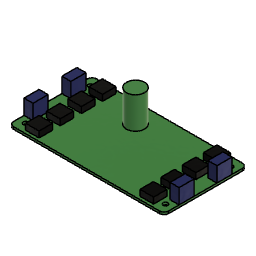
四路驱动模块 v2 (Autodesk Fusion 360 design; units mm, degrees)
Autodesk Fusion 360 part; units mm, degrees
sketch "草图1" plane through (0, 0, 0) normal (0, 0, 1) x (1, 0, 0)
  line L0 (3, 0) -> (100.2, 0)
  line L1 (103.2, 3) -> (103.2, 52.2)
  line L2 (100.2, 55.2) -> (3, 55.2)
  line L3 (0, 52.2) -> (0, 3)
  line L4 (-10, 27.6) -> (117.08, 27.6)
  line L5 (51.6, 65) -> (51.6, -15)
  circle A0 centre (5, 49.2) radius 1.6
  circle A1 centre (98.2, 49.2) radius 1.6
  circle A2 centre (5, 6) radius 1.6
  circle A3 centre (98.2, 6) radius 1.6
  arc A4 (3, 55.2) -> (0, 52.2) centre (3, 52.2) ccw
  arc A5 (103.2, 52.2) -> (100.2, 55.2) centre (100.2, 52.2) ccw
  arc A6 (100.2, 0) -> (103.2, 3) centre (100.2, 3) ccw
  arc A7 (0, 3) -> (3, 0) centre (3, 3) ccw
  point P0 (103.2, 0)
  point P1 (0, 55.2)
  dimension "d1" = 103.2
  dimension "d2" = 55.2
  dimension "d3" = 3.2
  dimension "d4" = 93.2
  dimension "d5" = 43.2
  dimension "d6" = 3
  constraint horizontal L0
  constraint vertical L1
  constraint horizontal L2
  constraint vertical L3
  constraint perpendicular L1 L4
  constraint perpendicular L2 L5
  constraint symmetric L1 L3 L5
  constraint symmetric L0 L2 L4
  constraint symmetric L5 A0 A1
  constraint symmetric L4 A0 A2
  constraint symmetric L4 A1 A3
  constraint coincident P1 L2
  constraint coincident P1 L3
  constraint tangent L2 A4
  constraint tangent L3 A4
  constraint tangent L1 A5
  constraint tangent L2 A5
  constraint equal A4 A5
  constraint coincident P0 L0
  constraint coincident P0 L1
  constraint tangent L0 A6
  constraint tangent L1 A6
  constraint equal A4 A6
  constraint tangent L0 A7
  constraint tangent L3 A7
  constraint equal A4 A7
  measures "d1" distance of origin P0
  measures "d2" distance of origin P1
  measures "d3" diameter of A0
  measures "d4" distance of A2.centre A3.centre
  measures "d5" distance of A0.centre A2.centre
  measures "d6" radius of A4
extrude "拉伸1" add sketch "草图1" along normal blind 1.5 makes body 1
sketch "草图2" plane through (0, 0, 1.5) normal (0, 0, 1) x (-1, 0, 0)
  circle A0 centre (-98.2, -6) radius 1.6
  circle A1 centre (-5, -49.2) radius 1.6
  circle A2 centre (-5, -6) radius 1.6
  circle A3 centre (-98.2, -49.2) radius 1.6
  arc A4 (0, -3) -> (-3, 0) centre (-3, -3) ccw
  line L0 (-3, 0) -> (-100.2, 0)
  arc A5 (-100.2, 0) -> (-103.2, -3) centre (-100.2, -3) ccw
  line L1 (-103.2, -3) -> (-103.2, -52.2)
  arc A6 (-103.2, -52.2) -> (-100.2, -55.2) centre (-100.2, -52.2) ccw
  line L2 (-100.2, -55.2) -> (-3, -55.2)
  arc A7 (-3, -55.2) -> (0, -52.2) centre (-3, -52.2) ccw
  line L3 (0, -52.2) -> (0, -3)
  line L4 (11.7384, -27.6) -> (-122.0621, -27.6)
  line L5 (-51.6, -62.4053) -> (-51.6, 35)
  line L6 (0, -45.2) -> (-6, -45.2)
  line L7 (-6, -45.2) -> (-6, -35.2)
  line L8 (-6, -35.2) -> (0, -35.2)
  line L9 (0, -35.2) -> (0, -45.2)
  line L10 (-97.2, -35.2) -> (-103.2, -35.2)
  line L11 (-103.2, -35.2) -> (-103.2, -45.2)
  line L12 (-103.2, -45.2) -> (-97.2, -45.2)
  line L13 (-97.2, -45.2) -> (-97.2, -35.2)
  line L14 (0, -10) -> (-6, -10)
  line L15 (-6, -10) -> (-6, -20)
  line L16 (0, -20) -> (0, -10)
  line L17 (-6, -20) -> (0, -20)
  line L18 (-97.2, -20) -> (-103.2, -20)
  line L19 (-103.2, -10) -> (-97.2, -10)
  line L20 (-97.2, -10) -> (-97.2, -20)
  line L21 (-103.2, -20) -> (-103.2, -10)
  dimension "d9" = 10
  dimension "d10" = 6
  dimension "d11" = 10
  constraint perpendicular L3 L4
  constraint vertical L5
  constraint symmetric L1 L3 L5
  constraint symmetric L0 L2 L4
  constraint horizontal L6
  constraint vertical L7
  constraint horizontal L8
  constraint vertical L9
  constraint coincident L3 L6.start
  constraint symmetric L5 L6.start L11.end
  constraint symmetric L5 L6.end L12.end
  constraint symmetric L5 L7.end L10.start
  constraint symmetric L5 L8.end L10.end
  constraint symmetric L4 L6.start L14.start
  constraint symmetric L4 L6.end L14.end
  constraint symmetric L4 L7.end L15.end
  constraint symmetric L4 L8.end L16.start
  constraint symmetric L4 L10.start L18.start
  constraint symmetric L4 L10.end L18.end
  constraint symmetric L4 L11.end L19.start
  constraint symmetric L4 L12.end L19.end
  measures "d9" distance of L6.start L8.end
  measures "d10" distance of L6.start L6.end
  measures "d11" distance of L2 L6
extrude "拉伸2" add sketch "草图2" along normal blind 10 separate body contours L3 L14 L15 L16 L17 | L3 L6 L7 L8 L9 | L1 L18 L19 L20 L21 | L1 L10 L11 L12 L13 makes body 2 at (0, 16.6667, 4.8333) makes body 3 at (97.2, 41.8667, 4.8333) makes body 4 at (0, 41.8667, 4.8333) makes body 5 at (97.2, 13.3333, 4.8333)
sketch "草图3" plane through (0, 0, 1.5) normal (0, 0, 1) x (-1, 0, 0)
  circle A0 centre (-98.2, -6) radius 1.6
  circle A1 centre (-5, -49.2) radius 1.6
  circle A2 centre (-5, -6) radius 1.6
  circle A3 centre (-98.2, -49.2) radius 1.6
  arc A4 (0, -3) -> (-3, 0) centre (-3, -3) ccw
  line L0 (-3, 0) -> (-100.2, 0)
  arc A5 (-100.2, 0) -> (-103.2, -3) centre (-100.2, -3) ccw
  line L1 (-103.2, -3) -> (-103.2, -52.2)
  arc A6 (-103.2, -52.2) -> (-100.2, -55.2) centre (-100.2, -52.2) ccw
  line L2 (-100.2, -55.2) -> (-3, -55.2)
  arc A7 (-3, -55.2) -> (0, -52.2) centre (-3, -52.2) ccw
  line L3 (0, -52.2) -> (0, -3)
  line L4 (8.1327, -27.6) -> (-117.8159, -27.6)
  line L5 (-51.6, -63.777) -> (-51.6, 13.1538)
  line L6 (-9, -53.2) -> (-18, -53.2)
  line L7 (-18, -53.2) -> (-18, -44.2)
  line L8 (-18, -44.2) -> (-9, -44.2)
  line L9 (-9, -44.2) -> (-9, -53.2)
  line L10 (-9, -39.2) -> (-18, -39.2)
  line L11 (-18, -39.2) -> (-18, -30.2)
  line L12 (-18, -30.2) -> (-9, -30.2)
  line L13 (-9, -30.2) -> (-9, -39.2)
  line L14 (-18, -11) -> (-9, -11)
  line L15 (-9, -2) -> (-18, -2)
  line L16 (-9, -11) -> (-9, -2)
  line L17 (-18, -2) -> (-18, -11)
  line L18 (-9, -16) -> (-18, -16)
  line L19 (-9, -25) -> (-9, -16)
  line L20 (-18, -16) -> (-18, -25)
  line L21 (-18, -25) -> (-9, -25)
  line L22 (-94.2, -53.2) -> (-85.2, -53.2)
  line L23 (-94.2, -44.2) -> (-94.2, -53.2)
  line L24 (-85.2, -53.2) -> (-85.2, -44.2)
  line L25 (-85.2, -44.2) -> (-94.2, -44.2)
  line L26 (-94.2, -39.2) -> (-85.2, -39.2)
  line L27 (-94.2, -30.2) -> (-94.2, -39.2)
  line L28 (-85.2, -39.2) -> (-85.2, -30.2)
  line L29 (-85.2, -30.2) -> (-94.2, -30.2)
  line L30 (-85.2, -25) -> (-94.2, -25)
  line L31 (-94.2, -25) -> (-94.2, -16)
  line L32 (-85.2, -16) -> (-85.2, -25)
  line L33 (-94.2, -16) -> (-85.2, -16)
  line L34 (-85.2, -11) -> (-94.2, -11)
  line L35 (-94.2, -11) -> (-94.2, -2)
  line L36 (-85.2, -2) -> (-85.2, -11)
  line L37 (-94.2, -2) -> (-85.2, -2)
  dimension "d14" = 9
  dimension "d15" = 9
  dimension "d16" = 9
  dimension "d17" = 9
  dimension "d18" = 2
  dimension "d19" = 16
  dimension "d20" = 9
  dimension "d21" = 9
  constraint perpendicular L1 L4
  constraint perpendicular L4 L5
  constraint symmetric L1 L3 L5
  constraint symmetric L0 L2 L4
  constraint horizontal L6
  constraint vertical L7
  constraint horizontal L8
  constraint vertical L9
  constraint horizontal L10
  constraint vertical L11
  constraint horizontal L12
  constraint vertical L13
  constraint symmetric L4 L6.start L15.start
  constraint symmetric L4 L6.end L15.end
  constraint symmetric L4 L7.end L14.start
  constraint symmetric L4 L8.end L14.end
  constraint symmetric L4 L10.start L18.start
  constraint symmetric L4 L10.end L18.end
  constraint symmetric L4 L11.end L20.end
  constraint symmetric L4 L12.end L19.start
  constraint symmetric L5 L6.start L22.start
  constraint symmetric L5 L6.end L22.end
  constraint symmetric L5 L7.end L24.end
  constraint symmetric L5 L8.end L23.start
  constraint symmetric L5 L10.start L26.start
  constraint symmetric L5 L10.end L26.end
  constraint symmetric L5 L11.end L28.end
  constraint symmetric L5 L12.end L27.start
  constraint symmetric L5 L14.start L34.start
  constraint symmetric L5 L14.end L34.end
  constraint symmetric L5 L15.start L35.end
  constraint symmetric L5 L15.end L36.start
  constraint symmetric L5 L18.start L31.end
  constraint symmetric L5 L18.end L32.start
  constraint symmetric L5 L19.start L30.end
  constraint symmetric L5 L20.end L30.start
  measures "d14" distance of L6.start L6.end
  measures "d15" distance of L6.end L7.end
  measures "d16" distance of L10.end L11.end
  measures "d17" distance of L11.end L12.end
  measures "d18" distance of L2 L6
  measures "d19" distance of L2 L10
  measures "d20" distance of L3 L9
  measures "d21" distance of L3 L13
extrude "拉伸3" add sketch "草图3" along normal blind 4 separate body contours L6 L7 L8 L9 | L10 L11 L12 L13 | L14 L15 L16 L17 | L18 L19 L20 L21 | L22 L23 L24 L25 | L26 L27 L28 L29 | L30 L31 L32 L33 | L34 L35 L36 L37 makes body 6 at (88.2, 33.2, 1.5) makes body 7 at (12, 36.2, 1.5) makes body 8 at (15, 22, 1.5) makes body 9 at (91.2, 19, 1.5) makes body 10 at (88.2, 47.2, 1.5) makes body 11 at (15, 50.2, 1.5) makes body 12 at (12, 8, 1.5) makes body 13 at (88.2, 8, 1.5)
sketch "草图4" plane through (0, 0, 1.5) normal (0, 0, 1) x (-1, 0, 0)
  circle A0 centre (-98.2, -6) radius 1.6
  circle A1 centre (-5, -49.2) radius 1.6
  circle A2 centre (-5, -6) radius 1.6
  circle A3 centre (-98.2, -49.2) radius 1.6
  arc A4 (0, -3) -> (-3, 0) centre (-3, -3) ccw
  line L0 (-3, 0) -> (-100.2, 0)
  arc A5 (-100.2, 0) -> (-103.2, -3) centre (-100.2, -3) ccw
  line L1 (-103.2, -3) -> (-103.2, -52.2)
  arc A6 (-103.2, -52.2) -> (-100.2, -55.2) centre (-100.2, -52.2) ccw
  line L2 (-100.2, -55.2) -> (-3, -55.2)
  arc A7 (-3, -55.2) -> (0, -52.2) centre (-3, -52.2) ccw
  line L3 (0, -52.2) -> (0, -3)
  circle A8 centre (-42, -42.2) radius 6
  dimension "d24" = 42
  dimension "d25" = 13
  dimension "d26" = 12
  measures "d24" distance of L3 A8.centre
  measures "d25" distance of L2 A8.centre
  measures "d26" diameter of A8
extrude "拉伸4" add sketch "草图4" along normal blind 21 separate body contours A8 makes body 14
sketch "草图5" plane through (0, 0, 1.5) normal (0, 0, 1) x (-1, 0, 0)
  circle A0 centre (-98.2, -6) radius 1.6
  circle A1 centre (-5, -49.2) radius 1.6
  circle A2 centre (-5, -6) radius 1.6
  circle A3 centre (-98.2, -49.2) radius 1.6
  arc A4 (0, -3) -> (-3, 0) centre (-3, -3) ccw
  line L0 (-3, 0) -> (-100.2, 0)
  arc A5 (-100.2, 0) -> (-103.2, -3) centre (-100.2, -3) ccw
  line L1 (-103.2, -3) -> (-103.2, -52.2)
  arc A6 (-103.2, -52.2) -> (-100.2, -55.2) centre (-100.2, -52.2) ccw
  line L2 (-100.2, -55.2) -> (-3, -55.2)
  arc A7 (-3, -55.2) -> (0, -52.2) centre (-3, -52.2) ccw
  line L3 (0, -52.2) -> (0, -3)
sketch "草图6" plane through (0, 0, 1.5) normal (0, 0, 1) x (1, 0, 0)
copy_body "实体->零部件1" bodies 1 removing the originals makes body 15 in component "Component'"
copy_body "实体->零部件2" bodies 2 removing the originals makes body 16 in component "Component''"
copy_body "实体->零部件3" bodies 3 removing the originals makes body 17 in component "Component'''"
copy_body "实体->零部件4" bodies 4 removing the originals makes body 18 in component "Component''''"
copy_body "实体->零部件5" bodies 5 removing the originals makes body 19 in component "Component'''''"
copy_body "实体->零部件6" bodies 6 removing the originals makes body 20 in component "Component''''''"
copy_body "实体->零部件7" bodies 7 removing the originals makes body 21 in component "Component'''''''"
copy_body "实体->零部件8" bodies 8 removing the originals makes body 22 in component "Component''''''''"
copy_body "实体->零部件9" bodies 9 removing the originals makes body 23 in component "Component'''''''''"
copy_body "实体->零部件10" bodies 10 removing the originals makes body 24 in component "Component''''''''''"
copy_body "实体->零部件11" bodies 11 removing the originals makes body 25 in component "Component'''''''''''"
copy_body "实体->零部件12" bodies 12 removing the originals makes body 26 in component "Component''''''''''''"
copy_body "实体->零部件13" bodies 13 removing the originals makes body 27 in component "Component'''''''''''''"
copy_body "实体->零部件14" bodies 14 removing the originals makes body 28 in component "Component''''''''''''''"
component "Component'" placed x (1, 0, 0) y (0, 1, 0) z (0, 0, 1) at (0, 0, 0)
component "Component''" placed x (1, 0, 0) y (0, 1, 0) z (0, 0, 1) at (0, 0, 0)
component "Component'''" placed x (1, 0, 0) y (0, 1, 0) z (0, 0, 1) at (0, 0, 0)
component "Component''''" placed x (1, 0, 0) y (0, 1, 0) z (0, 0, 1) at (0, 0, 0)
component "Component'''''" placed x (1, 0, 0) y (0, 1, 0) z (0, 0, 1) at (0, 0, 0)
component "Component''''''" placed x (1, 0, 0) y (0, 1, 0) z (0, 0, 1) at (0, 0, 0)
component "Component'''''''" placed x (1, 0, 0) y (0, 1, 0) z (0, 0, 1) at (0, 0, 0)
component "Component''''''''" placed x (1, 0, 0) y (0, 1, 0) z (0, 0, 1) at (0, 0, 0)
component "Component'''''''''" placed x (1, 0, 0) y (0, 1, 0) z (0, 0, 1) at (0, 0, 0)
component "Component''''''''''" placed x (1, 0, 0) y (0, 1, 0) z (0, 0, 1) at (0, 0, 0)
component "Component'''''''''''" placed x (1, 0, 0) y (0, 1, 0) z (0, 0, 1) at (0, 0, 0)
component "Component''''''''''''" placed x (1, 0, 0) y (0, 1, 0) z (0, 0, 1) at (0, 0, 0)
component "Component'''''''''''''" placed x (1, 0, 0) y (0, 1, 0) z (0, 0, 1) at (0, 0, 0)
component "Component''''''''''''''" placed x (1, 0, 0) y (0, 1, 0) z (0, 0, 1) at (0, 0, 0)
